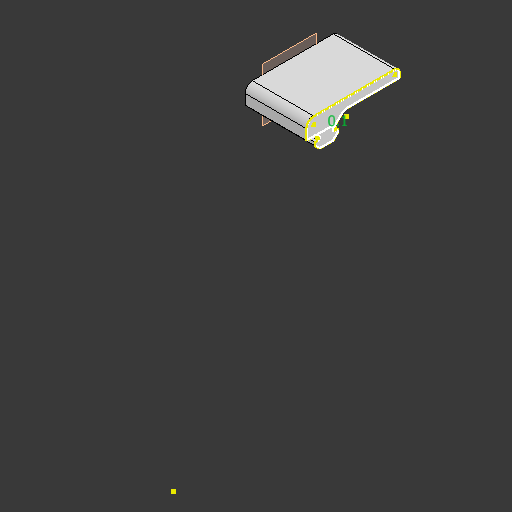
# Autodesk Inventor part: LED Holder
Saved by Autodesk Inventor 2023 (Build 270158000, 158)
## iProperties
Created: 2023-01-05
Part Number: LED Holder
Material: Generic
Document SubType Name: Modeling
Designer: alber
Density: 1 g/cm^3
Appearance: Default
Author: alber
Autodesk Inventor part; units mm, degrees
ref_plane "YZ Plane" through (0, 0, 0) normal (1, 0, 0) x (0, 1, 0)
ref_plane "XZ Plane" through (0, 0, 0) normal (0, 1, 0) x (-1, 0, 0)
ref_plane "XY Plane" through (0, 0, 0) normal (0, 0, 1) x (1, 0, 0)
ref_plane "Work Plane3" through (264.2728, 97.9235, -72.5028) normal (1, 0, 0) x (0, 1, 0)
sketch "Sketch1" plane through (264.2728, 97.9235, -72.5028) normal (1, 0, 0) x (0, 1, 0)
  line L0 (-1.8, 13.4828) -> (-1.8, 15.2101) projected
  line L1 (-1.8, 15.2101) -> (-3.8, 15.2101) projected
  line L2 (-3.8, 15.2101) -> (-6, 13.0101) projected
  line L3 (-6, 13.0101) -> (-6, 10.5) projected
  line L4 (-6, 9.5) -> (-6, 6.9899) projected
  line L5 (-6, 6.9899) -> (-3.8, 4.7899) projected
  line L6 (-3.8, 4.7899) -> (-1.8, 4.7899) projected
  line L7 (-1.8, 4.7899) -> (-1.8, 6.5172) projected
  line L8 (-6, 9.5) -> (-6, 10.5)
  line L9 (-0.0586, 14.7414) -> (-1.4586, 13.3414) projected
  arc A0 (-1.8, 13.4828) -> (-1.4586, 13.3414) centre (-1.6, 13.4828) ccw projected
  arc A1 (-1.4586, 6.6586) -> (-1.8, 6.5172) centre (-1.6, 6.5172) ccw projected
  line L10 (-1.4586, 6.6586) -> (-0.0586, 5.2586) projected
  line L11 (3.2, 2.7071) -> (-1.105, 7.0121)
  arc A2 (-1.105, 7.0121) -> (-2.3, 6.5172) centre (-1.6, 6.5172) ccw
  line L12 (-2.3, 6.5172) -> (-2.3, 5.2899)
  line L13 (-2.3, 5.2899) -> (-3.5929, 5.2899)
  line L14 (-3.5929, 5.2899) -> (-5.5, 7.1971)
  line L15 (-5.5, 7.1971) -> (-5.5, 9.5)
  line L16 (-5.5, 9.5) -> (-5.5, 10.5)
  line L17 (-5.5, 10.5) -> (-5.5, 12.8029)
  line L18 (-5.5, 12.8029) -> (-3.5929, 14.7101)
  line L19 (-3.5929, 14.7101) -> (-2.3, 14.7101)
  line L20 (-2.3, 14.7101) -> (-2.3, 13.4828)
  arc A3 (-2.3, 13.4828) -> (-1.105, 12.9879) centre (-1.6, 13.4828) ccw
  arc A4 (-0.2, 0) -> (0, 0.2) centre (-0.2, 0.2) ccw projected
  line L21 (0, 0.2) -> (0, 5.1172) projected
  arc A5 (0, 5.1172) -> (-0.0586, 5.2586) centre (-0.2, 5.1172) ccw projected
  line L22 (-1.4586, 6.6586) -> (-0.0586, 5.2586) projected
  arc A6 (-1.4586, 6.6586) -> (-1.8, 6.5172) centre (-1.6, 6.5172) ccw projected
  line L23 (-1.8, 4.7899) -> (-1.8, 6.5172) projected
  line L24 (-3.8, 4.7899) -> (-1.8, 4.7899) projected
  line L25 (-6, 6.9899) -> (-3.8, 4.7899) projected
  line L26 (-6, 9.5) -> (-6, 6.9899) projected
  line L27 (-6.5, 10) -> (-6, 9.5) projected
  line L28 (-6, 10.5) -> (-6.5, 10) projected
  line L29 (-6, 13.0101) -> (-6, 10.5) projected
  line L30 (-3.8, 15.2101) -> (-6, 13.0101) projected
  line L31 (-1.8, 15.2101) -> (-3.8, 15.2101) projected
  line L32 (-1.8, 13.4828) -> (-1.8, 15.2101) projected
  arc A7 (-1.8, 13.4828) -> (-1.4586, 13.3414) centre (-1.6, 13.4828) ccw projected
  line L33 (-0.0586, 14.7414) -> (-1.4586, 13.3414) projected
  arc A8 (-0.0586, 14.7414) -> (0, 14.8828) centre (-0.2, 14.8828) ccw projected
  line L34 (0, 14.8828) -> (0, 19.8) projected
  arc A9 (0, 19.8) -> (-0.2, 20) centre (-0.2, 19.8) ccw projected
  line L35 (-0.2, 20) -> (-5.1172, 20) projected
  arc A10 (-5.1172, 20) -> (-5.2586, 19.9414) centre (-5.1172, 19.8) ccw projected
  line L36 (-6.6586, 18.5414) -> (-5.2586, 19.9414) projected
  arc A11 (-6.6586, 18.5414) -> (-6.5172, 18.2) centre (-6.5172, 18.4) ccw projected
  line L37 (-4.7899, 18.2) -> (-6.5172, 18.2) projected
  line L38 (-4.7899, 16.2) -> (-4.7899, 18.2) projected
  line L39 (-6.9899, 14) -> (-4.7899, 16.2) projected
  line L40 (-9.5, 14) -> (-6.9899, 14) projected
  line L41 (-10, 13.5) -> (-9.5, 14) projected
  line L42 (-10.5, 14) -> (-10, 13.5) projected
  line L43 (-13.0101, 14) -> (-10.5, 14) projected
  line L44 (-15.2101, 16.2) -> (-13.0101, 14) projected
  line L45 (-15.2101, 18.2) -> (-15.2101, 16.2) projected
  line L46 (-13.4828, 18.2) -> (-15.2101, 18.2) projected
  arc A12 (-13.4828, 18.2) -> (-13.3414, 18.5414) centre (-13.4828, 18.4) ccw projected
  line L47 (-14.7414, 19.9414) -> (-13.3414, 18.5414) projected
  arc A13 (-14.7414, 19.9414) -> (-14.8828, 20) centre (-14.8828, 19.8) ccw projected
  line L48 (-14.8828, 20) -> (-19.8, 20) projected
  arc A14 (-19.8, 20) -> (-20, 19.8) centre (-19.8, 19.8) ccw projected
  line L49 (-20, 14.8828) -> (-20, 19.8) projected
  arc A15 (-20, 14.8828) -> (-19.9414, 14.7414) centre (-19.8, 14.8828) ccw projected
  line L50 (-18.5414, 13.3414) -> (-19.9414, 14.7414) projected
  arc A16 (-18.5414, 13.3414) -> (-18.2, 13.4828) centre (-18.4, 13.4828) ccw projected
  line L51 (-18.2, 15.2101) -> (-18.2, 13.4828) projected
  line L52 (-16.2, 15.2101) -> (-18.2, 15.2101) projected
  line L53 (-14, 13.0101) -> (-16.2, 15.2101) projected
  line L54 (-14, 10.5) -> (-14, 13.0101) projected
  line L55 (-13.5, 10) -> (-14, 10.5) projected
  line L56 (-14, 9.5) -> (-13.5, 10) projected
  line L57 (-14, 6.9899) -> (-14, 9.5) projected
  line L58 (-16.2, 4.7899) -> (-14, 6.9899) projected
  line L59 (-18.2, 4.7899) -> (-16.2, 4.7899) projected
  line L60 (-18.2, 6.5172) -> (-18.2, 4.7899) projected
  arc A17 (-18.2, 6.5172) -> (-18.5414, 6.6586) centre (-18.4, 6.5172) ccw projected
  line L61 (-19.9414, 5.2586) -> (-18.5414, 6.6586) projected
  arc A18 (-19.9414, 5.2586) -> (-20, 5.1172) centre (-19.8, 5.1172) ccw projected
  line L62 (-20, 0.2) -> (-20, 5.1172) projected
  arc A19 (-20, 0.2) -> (-19.8, 0) centre (-19.8, 0.2) ccw projected
  line L63 (-14.8828, 0) -> (-19.8, 0) projected
  arc A20 (-14.8828, 0) -> (-14.7414, 0.0586) centre (-14.8828, 0.2) ccw projected
  line L64 (-13.3414, 1.4586) -> (-14.7414, 0.0586) projected
  arc A21 (-13.3414, 1.4586) -> (-13.4828, 1.8) centre (-13.4828, 1.6) ccw projected
  line L65 (-15.2101, 1.8) -> (-13.4828, 1.8) projected
  line L66 (-15.2101, 3.8) -> (-15.2101, 1.8) projected
  line L67 (-13.0101, 6) -> (-15.2101, 3.8) projected
  line L68 (-10.5, 6) -> (-13.0101, 6) projected
  line L69 (-10, 6.5) -> (-10.5, 6) projected
  line L70 (-9.5, 6) -> (-10, 6.5) projected
  line L71 (-6.9899, 6) -> (-9.5, 6) projected
  line L72 (-4.7899, 3.8) -> (-6.9899, 6) projected
  line L73 (-4.7899, 1.8) -> (-4.7899, 3.8) projected
  line L74 (-6.5172, 1.8) -> (-4.7899, 1.8) projected
  arc A22 (-6.5172, 1.8) -> (-6.6586, 1.4586) centre (-6.5172, 1.6) ccw projected
  line L75 (-5.2586, 0.0586) -> (-6.6586, 1.4586) projected
  arc A23 (-5.2586, 0.0586) -> (-5.1172, 0) centre (-5.1172, 0.2) ccw projected
  line L76 (-0.2, 0) -> (-5.1172, 0) projected
  circle A24 centre (-10, 10) radius 2 projected
  line L77 (0, 5.9071) -> (0, 5.1172)
  line L78 (0.0036, 6) -> (0.0036, 5.9036)
  line L79 (3.2, 2.7071) -> (3.2, -20.1)
  line L80 (0.0036, -20.1) -> (0, -20.1)
  line L81 (0, 1.6971) -> (0, 1.8)
  line L82 (3.2, -20.1) -> (7.2, -20.1)
  line L83 (7.2, -20.1) -> (7.2, 4.9)
  line L84 (7.2, 4.9) -> (7.2, 15.9769)
  line L85 (0, 18.2) -> (7.2, 18.2)
  line L86 (7.2, 18.2) -> (7.2, 15.9769)
  line L87 (0, 18.2) -> (0.0036, 18.1982)
  line L88 (0, 14.8828) -> (0, 14.0929)
  line L89 (0, 14.0929) -> (-1.105, 12.9879)
  dimension "d0" = 0.5
  dimension "d10" = 4
  dimension "d11" = 3.2
  constraints: 48 end point, 11 point on line, 5 point on circle, 3 perpendicular, 3 vertical, 2 centre point, 2 horizontal, 2 parallel, 1 collinear, 10 other
  measures "d0" distance between parallel lines of L10 L11
  measures "d10" distance of L79.end L82.end
  measures "d11" distance between parallel lines of L21 L79
extrude "Extrusion1" add sketch "Sketch1" along normal blind 25 contours L34 L85 L86 L84 L83 L82 L79 L11 A2 L12 L13 L14 L15 L16 L17 L18 L19 L20 A3 L89 L88
fillet "Fillet1" radius 3 2 edges at (276.7728, 105.1235, -54.3028) (276.7728, 101.1235, -69.7956)
fillet "Fillet2" radius 2 1 edges at (276.7728, 105.1235, -92.6028)
sketch "Sketch4" plane through (289.2728, 97.9235, -72.5028) normal (1, 0, 0) x (0, 0, -1)
  point P0 (-72.5028, -97.9235)
sketch "Sketch5" plane through (289.2728, 97.9235, -72.5028) normal (1, 0, 0) x (0, 0, -1)
  arc A0 (20.1, 5.2) -> (18.1, 7.2) centre (18.1, 5.2) ccw projected
  line L0 (18.1, 7.2) -> (-15.2, 7.2) projected
  arc A1 (-15.2, 7.2) -> (-18.2, 4.2) centre (-15.2, 4.2) ccw projected
  line L1 (-18.2, 4.2) -> (-18.2, 0) projected
  line L2 (-18.2, 0) -> (-14.0929, 0) projected
  line L3 (-14.0929, 0) -> (-12.9879, -1.105) projected
  arc A2 (-13.4828, -2.3) -> (-12.9879, -1.105) centre (-13.4828, -1.6) ccw projected
  line L4 (-13.4828, -2.3) -> (-14.7101, -2.3) projected
  line L5 (-14.7101, -2.3) -> (-14.7101, -3.5929) projected
  line L6 (-14.7101, -3.5929) -> (-12.8029, -5.5) projected
  line L7 (-12.8029, -5.5) -> (-7.1971, -5.5) projected
  line L8 (-7.1971, -5.5) -> (-5.2899, -3.5929) projected
  line L9 (-5.2899, -3.5929) -> (-5.2899, -2.3) projected
  line L10 (-5.2899, -2.3) -> (-6.5172, -2.3) projected
  arc A3 (-7.0121, -1.105) -> (-6.5172, -2.3) centre (-6.5172, -1.6) ccw projected
  line L11 (-7.0121, -1.105) -> (-3.5858, 2.3213) projected
  arc A4 (-1.4645, 3.2) -> (-3.5858, 2.3213) centre (-1.4645, 0.2) ccw projected
  line L12 (-1.4645, 3.2) -> (20.1, 3.2) projected
  line L13 (20.1, 3.2) -> (20.1, 5.2) projected
  line L14 (-14.0929, 0) -> (-5.9071, 0)
  line L15 (-3.6565, 2.392) -> (-7.0828, -1.0343)
  arc A5 (-7.0828, -1.0343) -> (-6.5172, -2.4) centre (-6.5172, -1.6) ccw
  line L16 (-6.5172, -2.4) -> (-5.3899, -2.4)
  line L17 (-5.3899, -2.4) -> (-5.3899, -3.5515)
  line L18 (-5.3899, -3.5515) -> (-7.2385, -5.4)
  line L19 (-7.2385, -5.4) -> (-12.7615, -5.4)
  line L20 (-12.7615, -5.4) -> (-14.6101, -3.5515)
  line L21 (-14.6101, -3.5515) -> (-14.6101, -2.4)
  line L22 (-14.6101, -2.4) -> (-13.4828, -2.4)
  arc A6 (-13.4828, -2.4) -> (-12.9172, -1.0343) centre (-13.4828, -1.6) ccw
  line L23 (-12.9172, -1.0343) -> (-14.0515, 0.1)
  line L24 (-14.0515, 0.1) -> (-18.1, 0.1)
  line L25 (-18.1, 0.1) -> (-18.1, 4.2)
  arc A7 (-15.2, 7.1) -> (-18.1, 4.2) centre (-15.2, 4.2) ccw
  line L26 (-15.2, 7.1) -> (18.1, 7.1)
  arc A8 (20, 5.2) -> (18.1, 7.1) centre (18.1, 5.2) ccw
  line L27 (20, 5.2) -> (20, 3.3)
  line L28 (20, 3.3) -> (-1.4645, 3.3)
  arc A9 (-1.4645, 3.3) -> (-3.6565, 2.392) centre (-1.4645, 0.2) ccw
  point P0 (-72.5028, -97.9235)
  dimension "d14" = 0.1
  constraints: 30 end point, 10 point on circle, 5 centre point, 1 horizontal, 1 point on line, 18 other
  measures "d14" distance between parallel lines of L11 L15
body "Solid1"
